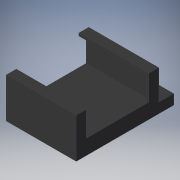
# Autodesk Inventor part: KVM Holder Left
Saved by Autodesk Inventor 2019 (Build 230136000, 136)
## iProperties
Created: 2021-02-17
Part Number: KVM Holder Left
Material: Generic
Document SubType Name: Modeling
Designer: dewanlab
Density: 1 g/cm^3
Appearance: Default
Author: dewanlab
Autodesk Inventor part; units mm, degrees
ref_plane "YZ Plane" through (0, 0, 0) normal (1, 0, 0) x (0, 1, 0)
ref_plane "XZ Plane" through (0, 0, 0) normal (0, 1, 0) x (-1, 0, 0)
ref_plane "XY Plane" through (0, 0, 0) normal (0, 0, 1) x (1, 0, 0)
sketch "Sketch1" plane through (0, 0, 0) normal (0, 1, 0) x (-1, 0, 0)
  line L0 (-44.45, -52.3875) -> (44.45, -52.3875)
  line L1 (44.45, -52.3875) -> (44.45, 52.3875)
  line L2 (44.45, 52.3875) -> (-44.45, 52.3875)
  line L3 (-44.45, 52.3875) -> (-44.45, -52.3875)
  line L4 (-44.45, -52.3875) -> (44.45, 52.3875) construction
  line L5 (44.45, -52.3875) -> (-44.45, 52.3875) construction
  point P0 (0, 0)
  dimension "d0" = 104.775
  dimension "d1" = 88.9
  constraints: 12 end point, 2 midpoint, 2 parallel, 1 horizontal, 1 perpendicular
  measures "d0" distance between parallel lines of L0 L2
  measures "d1" distance between parallel lines of L3 L1
extrude "Extrusion1" add sketch "Sketch1" along normal blind 12.7
sketch "Sketch2" plane through (0, 12.7, 0) normal (0, 1, 0) x (1, 0, 0)
  line L0 (44.45, 52.3875) -> (-44.45, 52.3875) projected
  line L1 (-44.45, 52.3875) -> (-44.45, -52.3875) projected
  line L2 (44.45, 52.3875) -> (-44.45, 52.3875)
  line L3 (-44.45, 52.3875) -> (-44.45, -52.3875)
  line L4 (-44.45, -52.3875) -> (44.45, -52.3875)
  line L5 (44.45, -52.3875) -> (44.45, 52.3875)
  point P0 (0, 0)
  dimension "d4" = 104.775
  constraints: 8 end point, 2 parallel, 1 horizontal, 1 perpendicular, 1 point on line
  measures "d4" distance between parallel lines of L0 L4
extrude "Extrusion2" add sketch "Sketch2" along normal blind 38.1
sketch "Sketch4" plane through (-44.45, 0, -52.3875) normal (-1, 0, 0) x (0, 0, 1)
  line L0 (101.6, 47.625) -> (3.175, 47.625)
  line L1 (3.175, 47.625) -> (3.175, 12.7)
  line L2 (3.175, 12.7) -> (101.6, 12.7)
  line L3 (101.6, 12.7) -> (101.6, 47.625)
  line L4 (0, 0) -> (0, 50.8) projected
  line L5 (0, 50.8) -> (104.775, 50.8) projected
  line L6 (104.775, 12.7) -> (104.775, 50.8)
  line L7 (0, 0) -> (104.775, 0) projected
  point P0 (52.3875, 0)
  dimension "d11" = 3.175
  dimension "d12" = 3.175
  dimension "d14" = 12.7
  dimension "d33" = 3.175
  constraints: 10 end point, 2 parallel, 1 horizontal, 1 perpendicular
  measures "d11" distance between parallel lines of L4 L1
  measures "d12" distance between parallel lines of L5 L0
  measures "d14" distance between parallel lines of L7 L2
  measures "d33" distance between parallel lines of L6 L3
extrude "Extrusion3" cut sketch "Sketch4" against normal blind 85.725
sketch "Sketch5" plane through (0, 50.8, 0) normal (0, 1, 0) x (1, 0, 0)
  line L0 (-44.45, 52.3875) -> (-44.45, -52.3875) projected
  line L1 (44.45, -52.3875) -> (44.45, 52.3875) projected
  line L2 (-44.45, -39.6875) -> (44.45, -39.6875)
  line L3 (44.45, -39.6875) -> (44.45, 39.6875)
  line L4 (44.45, 39.6875) -> (-44.45, 39.6875)
  line L5 (-44.45, 39.6875) -> (-44.45, -39.6875)
  line L6 (44.45, 52.3875) -> (-44.45, 52.3875) projected
  line L7 (-44.45, -52.3875) -> (44.45, -52.3875) projected
  point P0 (0, 0)
  dimension "d17" = 12.7
  dimension "d18" = 12.7
  constraints: 8 end point, 2 parallel, 2 point on line, 1 horizontal, 1 perpendicular
  measures "d17" distance between parallel lines of L6 L4
  measures "d18" distance between parallel lines of L2 L7
extrude "Extrusion4" cut sketch "Sketch5" against normal blind 31.75 contours L4 L1 L2 L0
sketch "Sketch7" plane through (44.45, 0, -52.3875) normal (0, 0, -1) x (-1, 0, 0)
  line L0 (88.9, 0) -> (0, 0) projected
  line L1 (0, 0) -> (0, 50.8) projected
  line L2 (88.9, 0) -> (0, 0)
  line L3 (0, 0) -> (0, 12.7)
  line L4 (0, 12.7) -> (88.9, 12.7)
  line L5 (88.9, 12.7) -> (88.9, 0)
  point P0 (44.45, 0)
  dimension "d30" = 12.7
  constraints: 8 end point, 2 parallel, 1 horizontal, 1 perpendicular, 1 point on line
  measures "d30" distance between parallel lines of L0 L4
extrude "Extrusion5" add sketch "Sketch7" along normal blind 19.05
sketch "Sketch8" plane through (-44.45, 12.7, -52.3875) normal (0, 1, 0) x (1, 0, 0)
  line L0 (0, 0) -> (0, 19.05) projected
  line L1 (88.9, 0) -> (88.9, 19.05) projected
  point P0 (44.45, -52.3875)
  point P1 (19.05, 10.5709)
  point P2 (69.85, 10.5709)
  dimension "d34" = 50.8
  dimension "d36" = 19.05
  measures "d34" distance of point (69.85, 10.571) point (19.05, 10.571)
  measures "d36" distance from line of L1 point (69.85, 10.571)
hole "Hole2" at (-25.4, 12.7, -62.9584) at (25.4, 12.7, -62.9584) direction (0, -1, 0) diameter 6.7564 end through all clearance for "Flat Head Machine Screw (82)" size "1/4" standard "Ansi Unified Screw Threads"
body "Solid1"
